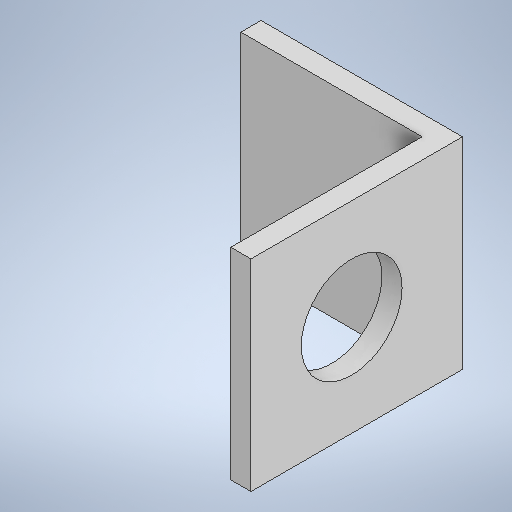
# Autodesk Inventor part: Holder for Main_Shaft
Saved by Autodesk Inventor 2025.2 (Build 292293000, 293)
## iProperties
Created: 2025-02-16
Part Number: Holder for Main_Shaft
Material: Generic
Document SubType Name: Modeling
Designer: shiva
Density: 1 g/cm^3
Appearance: Default
Author: shiva
Autodesk Inventor part; units mm, degrees
ref_plane "YZ Plane" through (0, 0, 0) normal (1, 0, 0) x (0, 1, 0)
ref_plane "XZ Plane" through (0, 0, 0) normal (0, 1, 0) x (-1, 0, 0)
ref_plane "XY Plane" through (0, 0, 0) normal (0, 0, 1) x (1, 0, 0)
sketch "Sketch1" plane through (0, 0, 0) normal (0, 0, 1) x (1, 0, 0)
  line L0 (-10, 10) -> (10, 10)
  line L1 (10, 10) -> (10, -10)
  line L2 (10, -10) -> (-10, -10)
  line L3 (-10, -10) -> (-10, 10)
  line L4 (-10, 10) -> (10, -10) construction
  line L5 (10, 10) -> (-10, -10) construction
  point P0 (0, 0)
  dimension "d0" = 20
  dimension "d1" = 20
  constraints: 12 end point, 2 midpoint, 2 parallel, 1 horizontal, 1 perpendicular
  measures "d0" distance of L1.end L2.end
  measures "d1" distance of L0.end L1.end
extrude "Extrusion1" add sketch "Sketch1" along normal blind 2
sketch "Sketch2" plane through (0, 0, 2) normal (0, 0, 1) x (1, 0, 0)
  line L0 (10, 10) -> (-10, 10) projected
  line L1 (-10, -10) -> (10, -10) projected
  line L2 (10, 10) -> (8, 10)
  line L3 (8, 10) -> (8, -10)
  line L4 (8, -10) -> (10, -10)
  line L5 (10, -10) -> (10, 10)
  point P0 (0, 0)
  dimension "d4" = 2
  constraints: 8 end point, 2 parallel, 1 horizontal, 1 perpendicular, 1 point on line
  measures "d4" distance of L4.end L3.end
extrude "Extrusion2" add sketch "Sketch2" along normal blind 19
sketch "Sketch3" plane through (10, -10, 0) normal (1, 0, 0) x (0, 0, -1)
  circle A0 centre (-11, 10) radius 5
  point P0 (0, 10)
  dimension "d7" = 10
  constraints: 1 centre point
  measures "d7" diameter of A0
extrude "Extrusion3" cut sketch "Sketch3" against normal up to surface (2 mm away)
body "Solid1"
